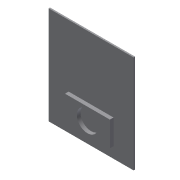
# Autodesk Inventor part: 02_Nanoscopy_Chip
Saved by Autodesk Inventor 2019 (Build 230136000, 136)
## iProperties
Created: 2017-12-13
Part Number: 02_Nanoscopy_Chip
Material: Generisch
Document SubType Name: Modeling
Designer: diederichbenedict
Density: 1 g/cm^3
Appearance: Vorgabe
Author: diederichbenedict
Autodesk Inventor part; units mm, degrees
ref_plane "YZ Plane" through (0, 0, 0) normal (1, 0, 0) x (0, 1, 0)
ref_plane "XZ Plane" through (0, 0, 0) normal (0, 1, 0) x (-1, 0, 0)
ref_plane "XY Plane" through (0, 0, 0) normal (0, 0, 1) x (1, 0, 0)
sketch "Skizze1" plane through (0, 0, 0) normal (0, 1, 0) x (-1, 0, 0)
  line L0 (0, 0) -> (23.3, 0)
  line L1 (23.3, 0) -> (23.3, 26.8)
  line L2 (23.3, 26.8) -> (0, 26.8)
  line L3 (0, 26.8) -> (0, 0)
  dimension "d0" = 23.3
  dimension "d1" = 26.8
  constraints: 8 end point, 2 parallel, 1 horizontal, 1 perpendicular
  measures "d0" distance of L2.end L1.end
  measures "d1" distance of L1.end L0.end
extrude "Extrusion1" add sketch "Skizze1" along normal blind 0.4
sketch "Skizze2" plane through (0, 0, 0) normal (0, -1, 0) x (1, 0, 0)
  line L0 (0, 0) -> (-23.3, 0) projected
  line L1 (0, 26.8) -> (0, 0) projected
  line L2 (-23.3, 26.8) -> (0, 26.8) projected
  line L3 (-23.3, 0) -> (-23.3, 26.8) projected
  line L4 (-17.8, 3) -> (-5.5, 3)
  line L5 (-5.5, 3) -> (-5.5, 9.8)
  line L6 (-5.5, 9.8) -> (-17.8, 9.8)
  line L7 (-17.8, 9.8) -> (-17.8, 3)
  dimension "d4" = 3
  dimension "d5" = 17
  dimension "d6" = 5.5
  dimension "d7" = 5.5
  constraints: 8 end point, 2 parallel, 1 horizontal, 1 perpendicular
  measures "d4" distance between parallel lines of L4 L0
  measures "d5" distance between parallel lines of L6 L2
  measures "d6" distance between parallel lines of L7 L3
  measures "d7" distance between parallel lines of L1 L5
extrude "Extrusion2" add sketch "Skizze2" along normal blind 1 contours L7 L6 L5 L4
sketch "Skizze3" plane through (0, -1, 0) normal (0, -1, 0) x (1, 0, 0)
  line L0 (-17.8, 3) -> (-5.5, 3) projected
  line L1 (-5.5, 3) -> (-5.5, 9.8) projected
  line L2 (-5.5, 9.8) -> (-17.8, 9.8) projected
  line L3 (-17.8, 9.8) -> (-17.8, 3) projected
  circle A0 centre (-11.65, 6.4) radius 2.9125
  point P0 (0, 0)
  constraints: 1 centre point
extrude "Extrusion3" cut sketch "Skizze3" against normal blind 1 contours A0
